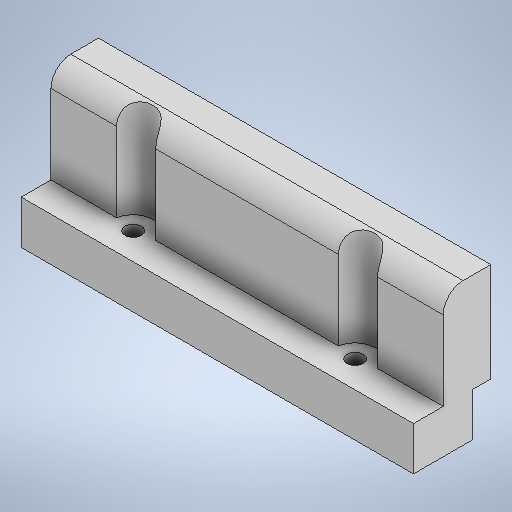
# Autodesk Inventor part: 13042026-15
Saved by Autodesk Inventor 2025.2 (Build 292293000, 293)
## iProperties
Created: 2026-05-27
Part Number: 13042026-15
Material: Generic
Document SubType Name: Modeling
Designer: Oski
Density: 1 g/cm^3
Appearance: Default
Author: Oski
Autodesk Inventor part; units mm, degrees
ref_plane "YZ Plane" through (0, 0, 0) normal (1, 0, 0) x (0, 1, 0)
ref_plane "XZ Plane" through (0, 0, 0) normal (0, 1, 0) x (-1, 0, 0)
ref_plane "XY Plane" through (0, 0, 0) normal (0, 0, 1) x (1, 0, 0)
sketch "Sketch1" plane through (0, 0, 0) normal (0, 0, 1) x (1, 0, 0)
  line L0 (-99, 11) -> (99, 11)
  line L1 (99, 11) -> (99, -11)
  line L2 (99, -11) -> (-99, -11)
  line L3 (-99, -11) -> (-99, 11)
  line L4 (-99, 11) -> (99, -11) construction
  line L5 (99, 11) -> (-99, -11) construction
  point P0 (0, 0)
  dimension "d0" = 22
  dimension "d1" = 198
  constraints: 12 end point, 2 midpoint, 2 parallel, 1 horizontal, 1 perpendicular
  measures "d0" distance of L0.end L1.end
  measures "d1" distance of L0.start L0.end
extrude "Extrusion1" add sketch "Sketch1" along normal blind 30
sketch "Sketch2" plane through (-99, 11, 0) normal (0, 1, 0) x (1, 0, 0)
  line L0 (0, 0) -> (0, -30) projected
  line L1 (0, -15) -> (198, -15)
  line L2 (198, -15) -> (198, 9)
  line L3 (198, 9) -> (0, 9)
  line L4 (0, 9) -> (0, -15)
  line L5 (198, 0) -> (198, -30) projected
  line L6 (198, 0) -> (0, 0) projected
  point P0 (99, 0)
  dimension "d4" = 9
  constraints: 8 end point, 2 midpoint, 2 parallel, 1 horizontal, 1 perpendicular
  measures "d4" distance between parallel lines of L3 L6
extrude "Extrusion2" add sketch "Sketch2" along normal blind 50
fillet "Fillet1" radius 10 1 edges at (0, 61, 15)
sketch "Sketch3" plane through (-99, 61, 0) normal (0, 1, 0) x (1, 0, 0)
  line L0 (0, -30) -> (198, -30) projected
  line L1 (198, 0) -> (198, -30) projected
  line L2 (155, -16.5) -> (198, -16.5) construction
  line L3 (43, -16.5) -> (0, -16.5) construction
  line L4 (0, -15) -> (0, -30) projected
  point P0 (99, 0)
  dimension "d17" = 13.5
  dimension "d19" = 13.5
  dimension "d21" = 112
  constraints: 4 end point, 2 collinear, 2 point on line, 1 horizontal, 1 perpendicular
  measures "d17" distance from line of L0 L3.start
  measures "d19" distance from line of L0 L2.start
  measures "d21" distance of L2.start L3.start
hole "Hole1" at (56, 61, 16.5) at (-56, 61, 16.5) direction (0, -1, 0) diameter 8.2 end through all counterbore diameter 20 counterbore depth 50
sketch "Sketch4" plane through (-99, -11, 0) normal (0, -1, 0) x (1, 0, 0)
  line L0 (198, 16.5) -> (0, 16.5) construction
  line L1 (0, 0) -> (0, 30) projected
  line L2 (198, 0) -> (198, 30) projected
  line L3 (0, 30) -> (198, 30) projected
  circle A0 centre (155, 16.5) radius 4.1
  circle A1 centre (155, 16.5) radius 4.1 projected
  line L4 (10.5, 25) -> (187.5, 25)
  line L5 (10.5, 8) -> (187.5, 8)
  arc A2 (187.5, 8) -> (187.5, 25) centre (187.5, 16.5) ccw
  arc A3 (10.5, 25) -> (10.5, 8) centre (10.5, 16.5) ccw
  line L6 (10.5, 16.5) -> (0, 16.5)
  line L7 (187.5, 16.5) -> (198, 16.5)
  point P0 (99, 0)
  point P1 (15, 16.5)
  point P2 (99, 16.5)
  point P3 (127, 16.5)
  point P4 (183, 16.5)
  point P5 (71, 16.5)
  dimension "d23" = 56
  dimension "d24" = 28
  dimension "d26" = 28
  dimension "d27" = 28
  dimension "d28" = 56
  dimension "d37" = 17
  dimension "d38" = 177
  constraints: 8 end point, 4 point on circle, 4 point on line, 3 centre point, 3 tangent, 2 concentric, 2 equal length, 2 horizontal, 2 perpendicular, 10 other
  measures "d23" distance of point (127, 16.5) point (183, 16.5)
  measures "d24" distance of point (99, 16.5) point (127, 16.5)
  measures "d26" distance of point (183, 16.5) A0.centre
  measures "d27" distance of point (71, 16.5) point (99, 16.5)
  measures "d28" distance of point (15, 16.5) point (71, 16.5)
  measures "d37" distance between parallel lines of L5 L4
  measures "d38" distance of L7.start L6.start
extrude "Extrusion3" cut sketch "Sketch4" against normal blind 10 contours A3 L4 A2 L5
sketch "Sketch5" plane through (-99, -1, 0) normal (0, -1, 0) x (1, 0, 0)
  circle A0 centre (43, 16.5) radius 10
  circle A1 centre (43, 16.5) radius 4.1 projected
  circle A2 centre (155, 16.5) radius 10
  circle A3 centre (155, 16.5) radius 4.1 projected
  circle A4 centre (43, 16.5) radius 4.1
  circle A5 centre (155, 16.5) radius 4.1
  point P0 (99, 0)
  dimension "d41" = 20
  constraints: 4 centre point, 3 equal radius, 2 coincident, 2 concentric
  measures "d41" diameter of A0
extrude "Extrusion4" add sketch "Sketch5" along normal blind 10
body "Solid1"
